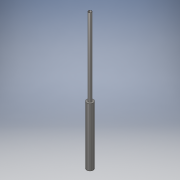
# Autodesk Inventor part: still pipe small.iam
Saved by Autodesk Inventor 2018 (Build 220112000, 112)
## iProperties
Created: 2019-02-25
Part Number: still pipe small.iam
Material: Stainless Steel
Document SubType Name: Modeling
Designer: Admin
Density: 8 g/cm^3
Appearance: Semi-Polished
Author: Admin
Autodesk Inventor part; units mm, degrees
ref_plane "YZ Plane" through (0, 0, 0) normal (1, 0, 0) x (0, 1, 0)
ref_plane "XZ Plane" through (0, 0, 0) normal (0, 1, 0) x (-1, 0, 0)
ref_plane "XY Plane" through (0, 0, 0) normal (0, 0, 1) x (1, 0, 0)
sketch "Sketch1" plane through (0, 0, 0) normal (0, 1, 0) x (-1, 0, 0)
  circle A0 centre (0, 0) radius 6.35
  circle A1 centre (0, 0) radius 5.715
  dimension "d0" = 12.7
  dimension "d1" = 0.635
  constraints: 2 centre point, 2 coincident
  measures "d0" diameter of A0
  measures "d1" radial gap between concentric circles of A0 A1
extrude "Extrusion1" add sketch "Sketch1" along normal blind 304.8
sketch "Sketch2" plane through (0, 0, 0) normal (0, -1, 0) x (1, 0, 0)
  circle A0 centre (0, 0) radius 6.35
  circle A1 centre (0, 0) radius 6.35 projected
  circle A2 centre (0, 0) radius 12.065
  dimension "d4" = 24.13
  constraints: 2 centre point, 2 coincident, 1 concentric
  measures "d4" diameter of A2
extrude "Extrusion2" add sketch "Sketch2" against normal blind 1.27
sketch "Sketch3" plane through (0, 1.27, 0) normal (0, 1, 0) x (1, 0, 0)
  circle A0 centre (0, 0) radius 12.065
  circle A1 centre (0, 0) radius 12.065 projected
  circle A2 centre (0, 0) radius 12.7
  dimension "d7" = 25.4
  constraints: 2 centre point, 2 coincident, 1 concentric
  measures "d7" diameter of A2
extrude "Extrusion3" add sketch "Sketch3" against normal blind 228.6
body "Solid1"
